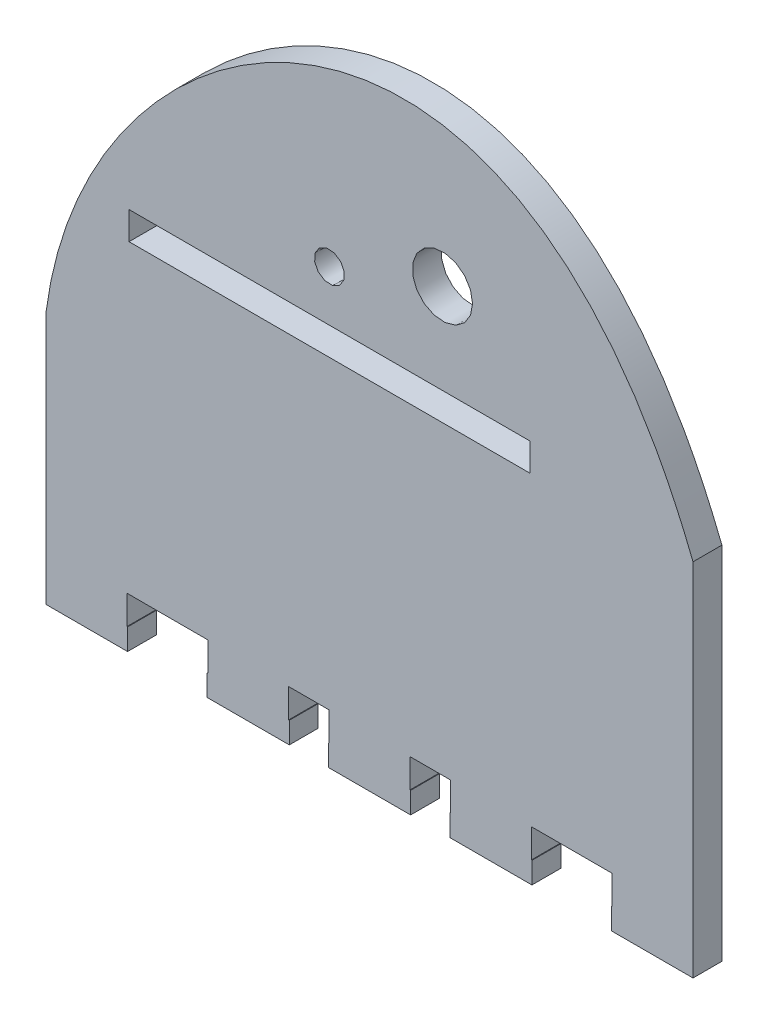
# Autodesk Inventor part: Part2
Saved by Autodesk Inventor 2016 (Build 200138000, 138)
## iProperties
Created: 2017-09-27
Part Number: Part2
Material: Generic
Document SubType Name: Modeling
Designer: student
Density: 1 g/cm^3
Appearance: Default
Author: student
Autodesk Inventor part; units mm, degrees
ref_plane "YZ Plane" through (0, 0, 0) normal (1, 0, 0) x (0, 1, 0)
ref_plane "XZ Plane" through (0, 0, 0) normal (0, 1, 0) x (-1, 0, 0)
ref_plane "XY Plane" through (0, 0, 0) normal (0, 0, 1) x (1, 0, 0)
sketch "Sketch1" plane through (0, 0, 0) normal (0, 0, 1) x (1, 0, 0)
  circle A0 centre (154.4814, -58.155) radius 3.048
  line L0 (114.3901, -106.0717) -> (114.3901, -96.2759)
  line L1 (179.8321, -69.61) -> (179.8321, -106.0717)
  line L2 (179.8321, -106.0717) -> (171.5883, -106.0717)
  line L3 (171.5883, -106.0717) -> (171.5883, -103.9127)
  line L4 (171.5883, -103.9127) -> (171.6518, -103.9127)
  line L5 (171.6518, -103.9127) -> (171.6518, -100.9917)
  line L6 (171.6518, -100.9917) -> (163.4716, -100.9917)
  line L7 (163.4716, -100.9917) -> (163.4716, -103.9127)
  line L8 (163.4716, -103.9127) -> (163.5351, -103.9127)
  line L9 (163.5351, -103.9127) -> (163.5351, -106.0717)
  line L10 (163.5351, -106.0717) -> (155.2278, -106.0717)
  line L11 (155.2278, -106.0717) -> (155.2278, -103.9127)
  line L12 (155.2278, -103.9127) -> (155.2913, -103.9127)
  line L13 (155.2913, -103.9127) -> (155.2913, -100.9917)
  line L14 (155.2913, -100.9917) -> (151.2012, -100.9917)
  line L15 (151.2012, -100.9917) -> (151.2012, -103.9127)
  line L16 (151.2012, -103.9127) -> (151.2647, -103.9127)
  line L17 (151.2647, -103.9127) -> (151.2647, -106.0717)
  line L18 (151.2647, -106.0717) -> (142.9575, -106.0717)
  line L19 (142.9575, -106.0717) -> (142.9575, -103.9127)
  line L20 (142.9575, -103.9127) -> (143.021, -103.9127)
  line L21 (143.021, -103.9127) -> (143.021, -100.9917)
  line L22 (143.021, -100.9917) -> (138.9308, -100.9917)
  line L23 (138.9308, -100.9917) -> (138.9308, -103.9127)
  line L24 (138.9308, -103.9127) -> (138.9943, -103.9127)
  line L25 (138.9943, -103.9127) -> (138.9943, -106.0717)
  line L26 (138.9943, -106.0717) -> (130.6871, -106.0717)
  line L27 (130.6871, -106.0717) -> (130.6871, -103.9127)
  line L28 (130.6871, -103.9127) -> (130.7506, -103.9127)
  line L29 (130.7506, -103.9127) -> (130.7506, -100.9917)
  line L30 (130.7506, -100.9917) -> (122.5703, -100.9917)
  line L31 (122.5703, -100.9917) -> (122.5703, -103.9127)
  line L32 (122.5703, -103.9127) -> (122.6338, -103.9127)
  line L33 (122.6338, -103.9127) -> (122.6338, -106.0717)
  line L34 (122.6338, -106.0717) -> (114.3901, -106.0717)
  line L35 (114.3901, -96.2759) -> (114.3901, -80.4177)
  arc A1 (141.9155, -61.1284) -> (144.1874, -61.1284) centre (143.0514, -62.1444) ccw
  arc A2 (144.1874, -61.1284) -> (141.9155, -61.1284) centre (143.0514, -62.1444) ccw
  spline S0 degree 3 poles (179.8321, -69.61) (160.956, -21.7418) (118.36, -49.0164) (114.3901, -80.4177) knots 0 0 0 0 1 1 1 1
  line L36 (163.3209, -70.0946) -> (122.7783, -70.0946)
  line L37 (163.3209, -70.0946) -> (163.3209, -67.2752)
  line L38 (122.7783, -67.2752) -> (163.3209, -67.2752)
  line L39 (122.7783, -70.0946) -> (122.7783, -67.2752)
  line L40 (143.0496, -67.2244) -> (142.9988, -67.2244) construction
  line L41 (142.9988, -67.2244) -> (143.0496, -67.2244) construction
  line L42 (143.0496, -70.1454) -> (143.1004, -70.1454) construction
  point P0 (0, 0)
  point P1 (152.6411, -43.7673)
  point P2 (128.8414, -53.0997)
  point P3 (142.9988, -67.2752)
  point P4 (143.0496, -70.0946)
  constraints: 86 end point, 4 point on circle, 3 centre point, 2 horizontal, 1 coincident, 1 midpoint, 1 point on line, 1 vertical, 4 other
extrude "Extrusion1" add sketch "Sketch1" along normal blind 2.921
body "Solid1"
